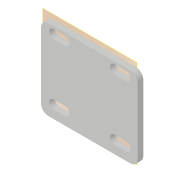
# Autodesk Inventor part: LiftLimitSwitchAdjuster
Saved by Autodesk Inventor 2018 (Build 220112000, 112)
## iProperties
Created: 2019-04-11
Part Number: LiftLimitSwitchAdjuster
Material: Generic
Document SubType Name: Modeling
Designer: ball
Density: 1 g/cm^3
Appearance: Default
Author: ball
Autodesk Inventor part; units mm, degrees
ref_plane "YZ Plane" through (0, 0, 0) normal (1, 0, 0) x (0, 1, 0)
ref_plane "XZ Plane" through (0, 0, 0) normal (0, 1, 0) x (-1, 0, 0)
ref_plane "XY Plane" through (0, 0, 0) normal (0, 0, 1) x (1, 0, 0)
ref_plane "Work Plane1" through (0, 0, 0) normal (0, 0, 1) x (1, 0, 0)
sketch "Sketch1" plane through (0, 0, 0) normal (0, 0, 1) x (1, 0, 0)
  line L0 (-17.78, -19.05) -> (17.78, -19.05) construction
  line L1 (19.05, -17.78) -> (19.05, 16.256) construction
  line L2 (-17.78, 16.764) -> (17.78, 16.764) construction
  circle A0 centre (-13.4704, -13.4704) radius 1.778 construction
  circle A1 centre (-13.4704, 13.4704) radius 1.778 construction
  circle A2 centre (13.4704, 13.4704) radius 1.778 construction
  circle A3 centre (13.4704, -13.4704) radius 1.778 construction
  line L3 (-19.05, -19.05) -> (23.6304, -19.05)
  line L4 (-13.4704, -13.4704) -> (19.05, -13.4704) construction
  line L5 (-13.4704, 13.4704) -> (19.05, 13.4704) construction
  line L6 (-13.4704, -13.4704) -> (-8.3904, -13.4704) construction
  line L7 (-13.4704, -15.4389) -> (-8.3904, -15.4389)
  line L8 (-8.3904, -11.5019) -> (-13.4704, -11.5019)
  arc A4 (-13.4704, -11.5019) -> (-13.4704, -15.4389) centre (-13.4704, -13.4704) ccw
  arc A5 (-8.3904, -15.4389) -> (-8.3904, -11.5019) centre (-8.3904, -13.4704) ccw
  line L9 (-13.4704, 13.4704) -> (-8.3904, 13.4704) construction
  line L10 (-13.4704, 11.5019) -> (-8.3904, 11.5019)
  line L11 (-8.3904, 15.4389) -> (-13.4704, 15.4389)
  arc A6 (-13.4704, 15.4389) -> (-13.4704, 11.5019) centre (-13.4704, 13.4704) ccw
  arc A7 (-8.3904, 11.5019) -> (-8.3904, 15.4389) centre (-8.3904, 13.4704) ccw
  line L12 (23.6304, 16.51) -> (23.6304, -19.05)
  line L13 (13.4704, -13.4704) -> (18.5504, -13.4704) construction
  line L14 (13.4704, -15.4389) -> (18.5504, -15.4389)
  line L15 (18.5504, -11.5019) -> (13.4704, -11.5019)
  arc A8 (13.4704, -11.5019) -> (13.4704, -15.4389) centre (13.4704, -13.4704) ccw
  arc A9 (18.5504, -15.4389) -> (18.5504, -11.5019) centre (18.5504, -13.4704) ccw
  line L16 (13.4704, 13.4704) -> (18.5504, 13.4704) construction
  line L17 (13.4704, 11.5019) -> (18.5504, 11.5019)
  line L18 (18.5504, 15.4389) -> (13.4704, 15.4389)
  arc A10 (13.4704, 15.4389) -> (13.4704, 11.5019) centre (13.4704, 13.4704) ccw
  arc A11 (18.5504, 11.5019) -> (18.5504, 15.4389) centre (18.5504, 13.4704) ccw
  line L19 (-19.05, 16.51) -> (23.6304, 16.51)
  line L20 (-19.05, 16.51) -> (-19.05, -19.05)
  point P0 (0, 0)
  point P1 (-10.9304, -13.4704)
  point P2 (-10.9304, 13.4704)
  point P3 (16.0104, -13.4704)
  point P4 (16.0104, 13.4704)
  dimension "d1" = 5.08
  dimension "d2" = 3.937
  dimension "d3" = 5.08
  dimension "d4" = 3.937
  dimension "d5" = 5.08
  dimension "d6" = 3.937
  dimension "d7" = 5.08
  dimension "d8" = 3.937
  dimension "d9" = 5.08
  constraints: 50 end point, 16 point on circle, 16 tangent, 12 centre point, 5 parallel, 5 point on line, 4 midpoint, 3 vertical, 2 horizontal, 13 other
  measures "d1" distance of L4.start L6.end
  measures "d2" diameter of A5
  measures "d3" distance of L5.start L9.end
  measures "d4" diameter of A7
  measures "d5" distance of L13.start L13.end
  measures "d6" diameter of A9
  measures "d7" distance of L16.start L16.end
  measures "d8" diameter of A11
  measures "d9" distance from line of L12 L13.end
extrude "Extrusion1" add sketch "Sketch1" along normal blind 2.54
fillet "Fillet1" radius 3.175 3 edges at (23.6304, 16.51, 1.27) (23.6304, -19.05, 1.27) (-19.05, -19.05, 1.27)
fillet "Fillet2" radius 3.175 1 edges at (-19.05, 16.51, 1.27)
body "Solid1"
